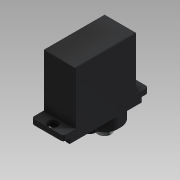
# Autodesk Inventor part: Corona
Saved by Autodesk Inventor 2014 (Build 180170000, 170)
## iProperties
Created: 2013-11-13
Part Number: Corona
Material: Générique
Document SubType Name: Modeling
Designer: Grégoire
Density: 1 g/cm^3
Appearance: Par défaut
Author: Grégoire
Autodesk Inventor part; units mm, degrees
ref_plane "YZ Plane" through (0, 0, 0) normal (1, 0, 0) x (0, 1, 0)
ref_plane "XZ Plane" through (0, 0, 0) normal (0, 1, 0) x (-1, 0, 0)
ref_plane "XY Plane" through (0, 0, 0) normal (0, 0, 1) x (1, 0, 0)
sketch "Esquisse1" plane through (0, 0, 0) normal (0, 0, 1) x (1, 0, 0)
  line L0 (0, 0) -> (12, 0)
  line L1 (12, 0) -> (12, 32)
  line L2 (12, 32) -> (0, 32)
  line L3 (0, 32) -> (0, 0)
  circle A0 centre (6, 30) radius 1.85
  line L4 (12, 16) -> (0, 16) construction
  circle A1 centre (6, 2) radius 1.85
  dimension "d0" = 32
  dimension "d1" = 12
  dimension "d2" = 28
  dimension "d3" = 3.7
  constraints: 10 end point, 2 centre point, 2 midpoint, 2 parallel, 1 horizontal, 1 perpendicular, 1 symmetric about line, 1 other
  measures "d0" distance of L0.end L1.end
  measures "d1" distance of L1.end L2.end
  measures "d2" distance of A1.centre A0.centre
  measures "d3" diameter of A0
extrude "Extrusion1" add sketch "Esquisse1" along normal blind 2
sketch "Esquisse2" plane through (0, 0, 2) normal (0, 0, 1) x (1, 0, 0)
  line L0 (0, 0) -> (12, 0) construction
  line L1 (12, 0) -> (12, 32) construction
  line L2 (12, 32) -> (0, 32) construction
  line L3 (0, 32) -> (0, 0) construction
  line L4 (0, 27.5) -> (12, 27.5)
  line L5 (12, 27.5) -> (12, 4.5)
  line L6 (12, 4.5) -> (0, 4.5)
  line L7 (0, 4.5) -> (0, 27.5)
  line L8 (6, 32) -> (6, 27.5) construction
  line L9 (6, 4.5) -> (6, 0) construction
  dimension "d6" = 23
  constraints: 12 end point, 4 midpoint, 2 parallel, 2 point on line, 1 collinear, 1 horizontal, 1 perpendicular
  measures "d6" distance of L4.end L5.end
extrude "Extrusion2" add sketch "Esquisse2" along normal blind 20
chamfer "Chanfrein1" distance 0.2 angle 45 4 edges at (6, 27.5, 22) (0, 16, 22) (12, 16, 22) (6, 4.5, 22)
sketch "Esquisse3" plane through (0, 0, 0) normal (0, 0, -1) x (-1, 0, 0)
  line L0 (0, 0) -> (-12, 0) construction
  line L1 (0, 32) -> (0, 0) construction
  line L2 (-12, 32) -> (0, 32) construction
  line L3 (-12, 0) -> (-12, 32) construction
  line L4 (-10.3, 27.45) -> (-1.7, 27.45)
  line L5 (0, 27.45) -> (0, 4.55)
  line L6 (-1.7, 4.55) -> (-10.3, 4.55)
  line L7 (-12, 4.55) -> (-12, 27.45)
  line L8 (-6, 32) -> (-6, 27.45) construction
  line L9 (-6, 4.55) -> (-6, 0) construction
  line L10 (-10.3, 27.45) -> (-10.3, 29.65)
  line L11 (-10.3, 29.65) -> (-12, 29.65)
  line L12 (-12, 29.65) -> (-12, 27.45)
  line L13 (-1.7, 27.45) -> (-1.7, 29.65)
  line L14 (-1.7, 29.65) -> (0, 29.65)
  line L15 (0, 29.65) -> (0, 27.45)
  line L16 (0, 16) -> (-12, 16) construction
  line L17 (-10.3, 4.55) -> (-10.3, 2.35)
  line L18 (-10.3, 2.35) -> (-12, 2.35)
  line L19 (-12, 2.35) -> (-12, 4.55)
  line L20 (-1.7, 4.55) -> (-1.7, 2.35)
  line L21 (-1.7, 2.35) -> (0, 2.35)
  line L22 (0, 2.35) -> (0, 4.55)
  dimension "d12" = 22.9
  dimension "d30" = 2.2
  dimension "d31" = 1.7
  constraints: 38 end point, 9 symmetric about line, 6 midpoint, 6 parallel, 3 collinear, 1 horizontal, 1 perpendicular
  measures "d12" distance between parallel lines of L6 L4
  measures "d30" distance of L4.start L10.end
  measures "d31" distance of L10.end L11.end
extrude "Extrusion3" add sketch "Esquisse3" along normal blind 2
sketch "Esquisse4" plane through (0, 0, -2) normal (0, 0, -1) x (-1, 0, 0)
  line L0 (-1.7, 27.45) -> (-10.3, 27.45) construction
  line L1 (-12, 29.65) -> (-12, 2.35) construction
  arc A0 (-3.0953, 16.2) -> (-8.9047, 16.2) centre (-6, 21.45) ccw
  line L2 (-6, 21.45) -> (-6, 27.45) construction
  arc A1 (-8.9047, 16.2) -> (-3.0953, 16.2) centre (-6, 15.45) ccw
  point P0 (0, 27.45)
  point P1 (-12, 27.45)
  point P2 (-12, 4.55)
  point P3 (0, 0)
  dimension "d15" = 12
  dimension "d16" = 6
  dimension "d17" = 6
  dimension "d18" = 22.5
  constraints: 5 point on circle, 2 centre point, 2 end point, 1 midpoint, 1 parallel
  measures "d15" diameter of A0
  measures "d16" distance of L2.start L2.end
  measures "d17" diameter of A1
  measures "d18" diameter of A0.start L0
extrude "Extrusion4" add sketch "Esquisse4" along normal blind 4
sketch "Esquisse5" plane through (0, 0, -6) normal (0, 0, -1) x (-1, 0, 0)
  arc A0 (-8.9047, 16.2) -> (-3.0953, 16.2) centre (-6, 15.45) ccw construction
  arc A1 (-3.0953, 16.2) -> (-8.9047, 16.2) centre (-6, 21.45) ccw construction
  arc A2 (-5.1092, 16.53) -> (-6.8908, 16.53) centre (-6, 21.45) ccw
  arc A3 (-6.8908, 16.53) -> (-5.1092, 16.53) centre (-6, 15.45) ccw
  point P0 (0, 0)
  dimension "d21" = 5
  dimension "d22" = 1.4
  constraints: 4 point on circle, 2 centre point, 2 coincident
  measures "d21" radius of A2
  measures "d22" radius of A3
extrude "Extrusion5" add sketch "Esquisse5" along normal blind 1
sketch "Esquisse6" plane through (0, 0, -7) normal (0, 0, -1) x (-1, 0, 0)
  arc A0 (-5.1092, 16.53) -> (-6.8908, 16.53) centre (-6, 21.45) ccw construction
  circle A1 centre (-6, 21.45) radius 2.5
  point P0 (0, 0)
  dimension "d25" = 5
  constraints: 1 centre point, 1 coincident
  measures "d25" diameter of A1
extrude "Extrusion6" add sketch "Esquisse6" along normal blind 3
fillet "Congé1" radius 0.3 8 edges at (12, 29.65, -1) (10.3, 29.65, -1) (1.7, 29.65, -1) (0, 29.65, -1) (10.3, 2.35, -1) (12, 2.35, -1) (1.7, 2.35, -1) (0, 2.35, -1)
fillet "Congé2" radius 1 4 edges at (0, 0, 1) (12, 0, 1) (0, 32, 1) (12, 32, 1)
chamfer "Chanfrein2" distance 0.2 angle 45 24 edges at (12, 25.4, -2) (11.9121, 29.5621, -2) (11.15, 29.65, -2) (10.3879, 29.5621, -2) (10.3, 28.4, -2) (12, 12.05, -2) (11.9121, 2.4379, -2) (11.15, 2.35, -2) (10.3879, 2.4379, -2) (10.3, 3.6, -2) (0, 12.05, -2) (0.0879, 2.4379, -2) (0.85, 2.35, -2) (1.6121, 2.4379, -2) (1.7, 3.6, -2) (0, 25.4, -2) (0.0879, 29.5621, -2) (0.85, 29.65, -2) (1.6121, 29.5621, -2) (1.7, 28.4, -2) (0, 27.5, 11.9) (0, 4.5, 11.9) (12, 4.5, 11.9) (12, 27.5, 11.9)
equation "\"d16\" = 0.5 * d15"
